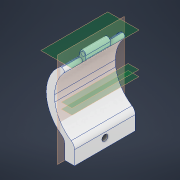
# Autodesk Inventor part: Hinge
Saved by Autodesk Inventor 2021 (Build 250183000, 183)
## iProperties
Created: 2021-05-17
Part Number: Hinge
Material: Aluminum 6061
Document SubType Name: Modeling
Designer: chick
Density: 2.7 g/cm^3
Appearance: Aluminum - Flat
Mass: 500.437 g
Surface Area: 374.372 cm^2
Volume: 185.347 cm^3
Author: chick
Autodesk Inventor part; units mm, degrees
ref_plane "XZ Plane" through (0, 0, 0) normal (0, 1, 0) x (-1, 0, 0)
ref_plane "XY Plane" through (0, 0, 0) normal (0, 0, 1) x (1, 0, 0)
sketch "Sketch1" plane through (0, 0, 0) normal (0, 0, 1) x (1, 0, 0)
  line L0 (7.1104, -129.7469) -> (23.1104, -129.7469)
  line L1 (7.1104, -129.7469) -> (7.1104, -99.7469)
  arc A0 (0, 0) -> (7.1104, -99.7469) centre (36.6375, -47.5152) ccw
  line L2 (0, 0) -> (12, 0)
  line L3 (23.1104, -129.7469) -> (23.1104, -99.7469)
  arc A1 (12, 0) -> (23.1104, -99.7469) centre (50.2435, -46.2324) ccw
  line L4 (-42.1677, 0) -> (65.6453, 0) projected
  line L5 (0, 25.9494) -> (0, -155.6963) projected
  point P0 (24.2536, -50)
  dimension "d1" = 100
  dimension "d2" = 60
  dimension "d3" = 30
  dimension "d5" = 12
  dimension "d37" = 60
  dimension "d38" = 30
  dimension "d43" = 12
  dimension "d44" = 16
  constraints: 8 end point, 4 point on circle, 2 centre point, 2 horizontal, 2 vertical, 1 point on line, 1 other
  measures "d1" distance of L1.end L2.start
  measures "d2" radius of A0
  measures "d3" distance of L0.start L1.end
  measures "d5" distance of L2.end L2.start
  measures "d37" radius of A1
  measures "d38" distance of L0.end L3.end
  measures "d44" distance of L0.start L0.end
extrude "Extrusion1" add sketch "Sketch1" along normal blind 100 contours L1 A0 L5 A1 L3 L0 | A0 L5 A1 | L2 A1 L5
sketch "Sketch2" plane through (0, 0, 100) normal (0, 0, 1) x (1, 0, 0)
  line L0 (12, 0) -> (0, 0) projected
  arc A0 (12, 0) -> (20, -100) centre (47.6245, -46.7376) ccw projected
  line L1 (12, 7) -> (12, 0)
  line L2 (12, 0) -> (2, 0)
  line L3 (2, 0) -> (2, 7)
  arc A1 (12, 7) -> (2, 7) centre (7, 7) ccw
  point P0 (2, 0)
  dimension "d11" = 7
  dimension "d12" = 5
  dimension "d13" = 10
  constraints: 6 end point, 2 point on circle, 1 centre point, 1 parallel, 1 other
  measures "d11" distance of L1.start L0.start
  measures "d12" radius of A1
  measures "d13" distance of L3.end L1.start
extrude "Extrusion2" add sketch "Sketch2" against normal blind 100
ref_plane "Work Plane1" through (7, 12, 100) normal (0, -1, 0) x (1, 0, 0)
sketch "Sketch3" plane through (7, 12, 100) normal (0, -1, 0) x (1, 0, 0)
  line L0 (5, 0) -> (5, -100) projected
  line L1 (5, -30) -> (5, 0)
  line L2 (5, 0) -> (-5, 0) projected
  line L3 (5, 0) -> (-5, 0)
  line L4 (-5, 0) -> (-5, -30)
  line L5 (-5, -100) -> (-5, 0) projected
  line L6 (5, -30) -> (-5, -30)
  point P0 (-7, -100)
  dimension "d41" = 30
  constraints: 8 end point, 2 collinear, 1 perpendicular, 1 point on line, 2 other
  measures "d41" distance between parallel lines of L2 L6
extrude "Extrusion3" cut sketch "Sketch3" along normal blind 12
sketch "Sketch4" plane through (7, 12, 100) normal (0, -1, 0) x (1, 0, 0)
  line L0 (-5.6828, -70) -> (8.2569, -70)
  line L1 (-5.6828, -100) -> (-5.6828, -70)
  line L2 (-5.6828, -100) -> (8.2569, -100)
  line L3 (-16.7565, -100) -> (16.1104, -100) projected
  line L4 (8.2569, -70) -> (8.2569, -100)
  point P0 (5, -100)
  dimension "d46" = 30
  constraints: 8 end point, 2 point on line, 1 horizontal, 1 perpendicular
  measures "d46" distance of L0.end L2.end
extrude "Extrusion4" cut sketch "Sketch4" along normal blind 12
sketch "Sketch5" plane through (7, 7, 30) normal (0, 0, -1) x (-1, 0, 0)
  circle A0 centre (0, 0) radius 3.5
  point P0 (7, -7)
  dimension "d22" = 7
  constraints: 1 centre point
  measures "d22" diameter of A0
extrude "Extrusion5" cut sketch "Sketch5" against normal blind 40
sketch "Sketch6" plane through (7.1104, -129.7469, 0) normal (-1, 0, 0) x (0, 0, 1)
  line L0 (0, 0) -> (100, 0) projected
  circle A0 centre (50, 15) radius 5
  point P0 (0, 129.7469)
  dimension "d25" = 15
  dimension "d26" = 10
  constraints: 1 centre point, 1 coincident
  measures "d25" distance from line of L0 point (50, 15)
  measures "d26" diameter of A0
hole "Hole1" at (7.1104, -114.7469, 50) direction (1, 0, 0) diameter 10 end through all
fillet "Fillet1" radius 3 1 edges at (0, 0, 50)
fillet "Fillet2" radius 4 2 edges at (12, 0, 85) (12, 0, 15)
fillet "Fillet3" radius 3 1 edges at (12, 0, 50)
fillet "Fillet4" radius 8 1 edges at (2, 0, 50)
fillet "Fillet5" radius 12 2 edges at (23.1104, -99.7469, 50) (7.1104, -99.7469, 50)
ref_plane "Work Plane2" through (7.1104, -44.7469, 0) normal (0, -1, 0) x (1, 0, 0)
ref_plane "Work Plane3" through (7.1104, -54.7469, 0) normal (0, -1, 0) x (1, 0, 0)
split_face "Split1"
split_face "Split2"
equation "\"d1\" = d6"
equation "\"d3\" = d7"
equation "\"d6\" = 100"
equation "\"d7\" = 30"
body "Solid1"
